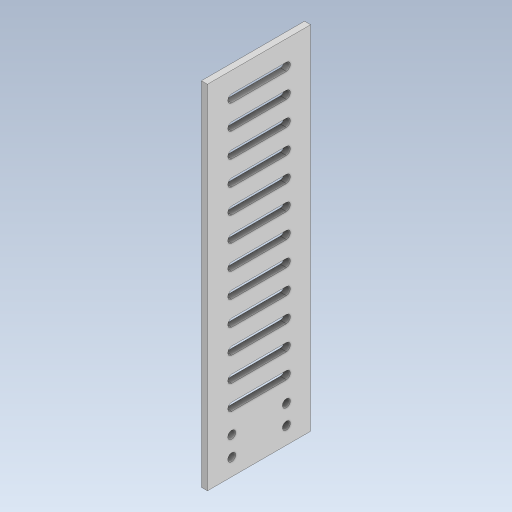
# Autodesk Inventor part: Wall Conyevor Depan
Saved by Autodesk Inventor 2023.5 (Build 275446000, 446)
## iProperties
Created: 2025-10-12
Part Number: Wall Conyevor Depan
Material: Generic
Document SubType Name: Modeling
Designer: Guntur
Density: 1 g/cm^3
Appearance: Default
Author: Guntur
## iProperties of the stored document Wall Conyevor Depan_3DPrint.ipt
Created: 2025-10-20
Part Number: Wall Conyevor Depan_3DPrint
Material: Generic
Document SubType Name: Modeling
Designer: Guntur
Density: 1 g/cm^3
Appearance: Default
Author: Guntur
Autodesk Inventor part; units mm, degrees
ref_plane "YZ Plane" through (0, 0, 0) normal (1, 0, 0) x (0, 1, 0)
ref_plane "XZ Plane" through (0, 0, 0) normal (0, 1, 0) x (-1, 0, 0)
ref_plane "XY Plane" through (0, 0, 0) normal (0, 0, 1) x (1, 0, 0)
sketch "Sketch1" plane through (0, 0, 0) normal (1, 0, 0) x (0, 1, 0)
  circle A0 centre (0, -22.5) radius 1.65
  circle A1 centre (-8, 0) radius 1.65
  circle A2 centre (-8, -22.5) radius 1.65
  line L0 (0, 0) -> (-15, 0)
  line L1 (-15, 0) -> (-15, -22.5)
  line L2 (0, -22.5) -> (0, 0)
  line L3 (-15, -22.5) -> (-15, -32.5)
  line L4 (-15, -32.5) -> (0, -32.5)
  line L5 (0, -32.5) -> (0, -22.5)
  line L6 (0, 0) -> (-15, 0)
  line L7 (-15, 0) -> (-15, 10)
  line L8 (-15, 10) -> (0, 10)
  line L9 (0, 10) -> (0, 0)
  line L10 (0, 10) -> (130, 10)
  line L11 (130, 10) -> (130, -32.5)
  line L12 (130, -32.5) -> (0, -32.5)
  line L13 (0, -32.5) -> (0, 10)
  line L14 (10, 0) -> (10, -22.5) construction
  line L15 (8.35, 0) -> (8.35, -22.5)
  line L16 (11.65, -22.5) -> (11.65, 0)
  arc A3 (11.65, 0) -> (8.35, 0) centre (10, 0) ccw
  arc A4 (8.35, -22.5) -> (11.65, -22.5) centre (10, -22.5) ccw
  line L17 (18.35, 0) -> (18.35, -22.5)
  line L18 (20, 0) -> (20, -22.5) construction
  line L19 (21.65, -22.5) -> (21.65, 0)
  arc A5 (21.65, 0) -> (18.35, 0) centre (20, 0) ccw
  arc A6 (18.35, -22.5) -> (21.65, -22.5) centre (20, -22.5) ccw
  line L20 (28.35, 0) -> (28.35, -22.5)
  line L21 (30, 0) -> (30, -22.5) construction
  line L22 (31.65, -22.5) -> (31.65, 0)
  arc A7 (31.65, 0) -> (28.35, 0) centre (30, 0) ccw
  arc A8 (28.35, -22.5) -> (31.65, -22.5) centre (30, -22.5) ccw
  line L23 (38.35, 0) -> (38.35, -22.5)
  line L24 (40, 0) -> (40, -22.5) construction
  line L25 (41.65, -22.5) -> (41.65, 0)
  arc A9 (41.65, 0) -> (38.35, 0) centre (40, 0) ccw
  arc A10 (38.35, -22.5) -> (41.65, -22.5) centre (40, -22.5) ccw
  line L26 (48.35, 0) -> (48.35, -22.5)
  line L27 (50, 0) -> (50, -22.5) construction
  line L28 (51.65, -22.5) -> (51.65, 0)
  arc A11 (51.65, 0) -> (48.35, 0) centre (50, 0) ccw
  arc A12 (48.35, -22.5) -> (51.65, -22.5) centre (50, -22.5) ccw
  line L29 (58.35, 0) -> (58.35, -22.5)
  line L30 (60, 0) -> (60, -22.5) construction
  line L31 (61.65, -22.5) -> (61.65, 0)
  arc A13 (61.65, 0) -> (58.35, 0) centre (60, 0) ccw
  arc A14 (58.35, -22.5) -> (61.65, -22.5) centre (60, -22.5) ccw
  line L32 (68.35, 0) -> (68.35, -22.5)
  line L33 (70, 0) -> (70, -22.5) construction
  line L34 (71.65, -22.5) -> (71.65, 0)
  arc A15 (71.65, 0) -> (68.35, 0) centre (70, 0) ccw
  arc A16 (68.35, -22.5) -> (71.65, -22.5) centre (70, -22.5) ccw
  line L35 (78.35, 0) -> (78.35, -22.5)
  line L36 (80, 0) -> (80, -22.5) construction
  line L37 (81.65, -22.5) -> (81.65, 0)
  arc A17 (81.65, 0) -> (78.35, 0) centre (80, 0) ccw
  arc A18 (78.35, -22.5) -> (81.65, -22.5) centre (80, -22.5) ccw
  line L38 (88.35, 0) -> (88.35, -22.5)
  line L39 (90, 0) -> (90, -22.5) construction
  line L40 (91.65, -22.5) -> (91.65, 0)
  arc A19 (91.65, 0) -> (88.35, 0) centre (90, 0) ccw
  arc A20 (88.35, -22.5) -> (91.65, -22.5) centre (90, -22.5) ccw
  line L41 (98.35, 0) -> (98.35, -22.5)
  line L42 (100, 0) -> (100, -22.5) construction
  line L43 (101.65, -22.5) -> (101.65, 0)
  arc A21 (101.65, 0) -> (98.35, 0) centre (100, 0) ccw
  arc A22 (98.35, -22.5) -> (101.65, -22.5) centre (100, -22.5) ccw
  line L44 (108.35, 0) -> (108.35, -22.5)
  line L45 (110, 0) -> (110, -22.5) construction
  line L46 (111.65, -22.5) -> (111.65, 0)
  arc A23 (111.65, 0) -> (108.35, 0) centre (110, 0) ccw
  arc A24 (108.35, -22.5) -> (111.65, -22.5) centre (110, -22.5) ccw
  line L47 (118.35, 0) -> (118.35, -22.5)
  line L48 (120, 0) -> (120, -22.5) construction
  line L49 (121.65, -22.5) -> (121.65, 0)
  arc A25 (121.65, 0) -> (118.35, 0) centre (120, 0) ccw
  arc A26 (118.35, -22.5) -> (121.65, -22.5) centre (120, -22.5) ccw
  circle A27 centre (0, 0) radius 1.65
  point P0 (10, -11.25)
  point P1 (20, -11.25)
  point P2 (30, -11.25)
  point P3 (40, -11.25)
  point P4 (50, -11.25)
  point P5 (60, -11.25)
  point P6 (70, -11.25)
  point P7 (80, -11.25)
  point P8 (90, -11.25)
  point P9 (100, -11.25)
  point P10 (110, -11.25)
  point P11 (120, -11.25)
  dimension "d1" = 3.3
  dimension "d3" = 3.3
  dimension "d5" = 3.3
  dimension "d6" = 10
  dimension "d7" = 10
  dimension "d9" = 3.3
  dimension "d13" = 10
  dimension "d20" = 15
  dimension "d22" = 7
  dimension "d23" = 7
  dimension "d24" = 8
  dimension "d25" = 3.3
  dimension "d26" = 8
  dimension "d27" = 8
  constraints: 124 end point, 48 point on circle, 28 centre point, 7 parallel, 4 horizontal, 4 tangent, 3 perpendicular, 3 point on line, 1 coincident, 1 midpoint, 1 vertical, 132 other
  measures "d1" diameter of A0
  measures "d3" diameter of A1
  measures "d5" diameter of A2
  measures "d6" distance of L3.end L3.start
  measures "d7" distance of L6.end L7.end
  measures "d9" diameter of A4
  measures "d13" distance of L15.start L17.start
  measures "d20" distance of L3.end L4.end
  measures "d22" distance from line of A2.centre L1
  measures "d23" distance from line of A1.centre L7
  measures "d24" distance of A1.centre point (0, 0)
  measures "d25" diameter of A27
  measures "d26" distance of A1.centre A27.centre
  measures "d27" distance of A2.centre A0.centre
extrude "Extrusion1" add sketch "Sketch1" along normal blind 2.5 contours A0 L2 A27 L9 L10 L11 L12 L5 | A0 L5 L4 L3 L1 L0 A1 A27 L2 | L0 A1 L7 L8 L9 A27
body "Solid1"
